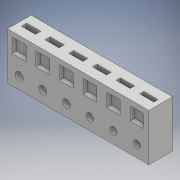
# Autodesk Inventor part: TOLERANCE_TEST
Saved by Autodesk Inventor 2017 (Build 210142000, 142)
## iProperties
Created: 2018-02-02
Part Number: TOLERANCE_TEST
Material: Generic
Document SubType Name: Modeling
Designer: Alex
Density: 1 g/cm^3
Appearance: Default
Author: Alex
Autodesk Inventor part; units mm, degrees
ref_plane "YZ Plane" through (0, 0, 0) normal (1, 0, 0) x (0, 1, 0)
ref_plane "XZ Plane" through (0, 0, 0) normal (0, 1, 0) x (-1, 0, 0)
ref_plane "XY Plane" through (0, 0, 0) normal (0, 0, 1) x (1, 0, 0)
sketch "Sketch1" plane through (0, 0, 0) normal (0, 1, 0) x (-1, 0, 0)
  line L0 (-30, 10) -> (30, 10)
  line L1 (30, 10) -> (30, -10)
  line L2 (30, -10) -> (-30, -10)
  line L3 (-30, -10) -> (-30, 10)
  point P0 (0, 0)
  point P1 (30, 0)
  point P2 (0, 10)
  dimension "d0" = 60
  dimension "d1" = 20
  constraints: 8 end point, 2 midpoint, 2 parallel, 1 horizontal, 1 horizontal alignment, 1 perpendicular, 1 vertical alignment
  measures "d0" distance of L0.start L0.end
  measures "d1" distance of L2.end L0.start
extrude "Extrusion1" add sketch "Sketch1" along normal blind 10
sketch "Sketch2" plane through (0, 10, 0) normal (0, 1, 0) x (1, 0, 0)
  line L0 (27.75, -7.75) -> (22.25, -7.75)
  line L1 (22.25, -7.75) -> (22.25, -2.25)
  line L2 (22.25, -2.25) -> (27.75, -2.25)
  line L3 (27.75, -2.25) -> (27.75, -7.75)
  line L4 (30, -10) -> (30, 10) projected
  line L5 (-30, -10) -> (30, -10) projected
  line L6 (12.2, -7.8) -> (17.8, -7.8)
  line L7 (17.8, -7.8) -> (17.8, -2.2)
  line L8 (17.8, -2.2) -> (12.2, -2.2)
  line L9 (12.2, -2.2) -> (12.2, -7.8)
  line L10 (2.15, -7.85) -> (7.85, -7.85)
  line L11 (7.85, -7.85) -> (7.85, -2.15)
  line L12 (7.85, -2.15) -> (2.15, -2.15)
  line L13 (2.15, -2.15) -> (2.15, -7.85)
  line L14 (-7.9, -7.9) -> (-2.1, -7.9)
  line L15 (-2.1, -7.9) -> (-2.1, -2.1)
  line L16 (-2.1, -2.1) -> (-7.9, -2.1)
  line L17 (-7.9, -2.1) -> (-7.9, -7.9)
  line L18 (-17.95, -7.95) -> (-12.05, -7.95)
  line L19 (-12.05, -7.95) -> (-12.05, -2.05)
  line L20 (-12.05, -2.05) -> (-17.95, -2.05)
  line L21 (-17.95, -2.05) -> (-17.95, -7.95)
  line L22 (-28, -8) -> (-22, -8)
  line L23 (-22, -8) -> (-22, -2)
  line L24 (-22, -2) -> (-28, -2)
  line L25 (-28, -2) -> (-28, -8)
  point P0 (0, 0)
  point P1 (-12.05, -5)
  point P2 (-7.9, -5)
  point P3 (-2.1, -5)
  point P4 (2.15, -5)
  point P5 (7.85, -5)
  point P6 (12.2, -5)
  point P7 (17.8, -5)
  point P8 (22.25, -5)
  point P9 (15, -7.8)
  point P10 (25, -7.75)
  point P11 (5, -7.85)
  point P12 (-5, -7.9)
  point P13 (-15, -7.95)
  point P14 (-25, -8)
  point P15 (-22, -5)
  point P16 (-17.95, -5)
  dimension "d9" = 5.5
  dimension "d10" = 5.6
  dimension "d11" = 5.7
  dimension "d12" = 5.8
  dimension "d13" = 5.9
  dimension "d14" = 10
  dimension "d15" = 10
  dimension "d16" = 10
  dimension "d17" = 10
  dimension "d18" = 5
  dimension "d19" = 6
  dimension "d20" = 10
  dimension "d65" = 5
  constraints: 48 end point, 16 midpoint, 12 parallel, 12 perpendicular, 6 horizontal, 5 horizontal alignment
  measures "d9" distance of L1.end L2.end
  measures "d10" distance of L7.end L8.end
  measures "d11" distance of L11.end L12.end
  measures "d12" distance of L15.end L16.end
  measures "d13" distance of L19.end L20.end
  measures "d14" horizontal distance of point (25, -7.75) point (15, -7.8)
  measures "d15" horizontal distance of point (15, -7.8) point (5, -7.85)
  measures "d16" horizontal distance of point (5, -7.85) point (-5, -7.9)
  measures "d17" horizontal distance of point (-5, -7.9) point (-15, -7.95)
  measures "d18" distance from line of L4 point (25, -7.75)
  measures "d19" distance of L23.end L24.end
  measures "d20" horizontal distance of point (-25, -8) point (-15, -7.95)
  measures "d65" distance from line of L5 point (22.25, -5)
extrude "Extrusion2" cut sketch "Sketch2" against normal blind 1.8
sketch "Sketch3" plane through (-30, 0, 10) normal (0, 0, 1) x (1, 0, 0)
  line L0 (2, 6.15) -> (8, 6.15)
  line L1 (8, 6.15) -> (8, 3.85)
  line L2 (8, 3.85) -> (2, 3.85)
  line L3 (2, 3.85) -> (2, 6.15)
  line L4 (12, 6.1) -> (18, 6.1)
  line L5 (18, 6.1) -> (18, 3.9)
  line L6 (18, 3.9) -> (12, 3.9)
  line L7 (12, 3.9) -> (12, 6.1)
  line L8 (22, 6.05) -> (28, 6.05)
  line L9 (28, 6.05) -> (28, 3.95)
  line L10 (28, 3.95) -> (22, 3.95)
  line L11 (22, 3.95) -> (22, 6.05)
  line L12 (32, 6) -> (38, 6)
  line L13 (38, 6) -> (38, 4)
  line L14 (38, 4) -> (32, 4)
  line L15 (32, 4) -> (32, 6)
  line L16 (42, 5.95) -> (48, 5.95)
  line L17 (48, 5.95) -> (48, 4.05)
  line L18 (48, 4.05) -> (42, 4.05)
  line L19 (42, 4.05) -> (42, 5.95)
  line L20 (52, 5.9) -> (58, 5.9)
  line L21 (58, 5.9) -> (58, 4.1)
  line L22 (58, 4.1) -> (52, 4.1)
  line L23 (52, 4.1) -> (52, 5.9)
  line L24 (60, 0) -> (60, 10) projected
  point P0 (30, 0)
  point P1 (55, 5.9)
  point P2 (45, 5.95)
  point P3 (35, 6)
  point P4 (25, 6.05)
  point P5 (15, 6.1)
  point P6 (5, 6.15)
  point P7 (8, 5)
  point P8 (12, 5)
  point P9 (18, 5)
  point P10 (22, 5)
  point P11 (28, 5)
  point P12 (32, 5)
  point P13 (38, 5)
  point P14 (42, 5)
  point P15 (48, 5)
  point P16 (52, 5)
  point P17 (58, 5)
  point P18 (60, 5)
  dimension "d23" = 6
  dimension "d24" = 1.8
  dimension "d25" = 5
  dimension "d26" = 10
  dimension "d27" = 10
  dimension "d28" = 10
  dimension "d29" = 10
  dimension "d30" = 10
  dimension "d31" = 1.9
  dimension "d32" = 2
  dimension "d33" = 2.1
  dimension "d34" = 2.2
  dimension "d35" = 2.3
  constraints: 48 end point, 18 midpoint, 17 parallel, 6 horizontal, 6 horizontal alignment, 6 perpendicular
  measures "d23" distance of L20.start L20.end
  measures "d24" distance of L20.end L21.end
  measures "d25" distance from line of point (55, 5.9) L24
  measures "d26" horizontal distance of point (55, 5.9) point (45, 5.95)
  measures "d27" horizontal distance of point (45, 5.95) point (35, 6)
  measures "d28" horizontal distance of point (35, 6) point (25, 6.05)
  measures "d29" horizontal distance of point (25, 6.05) point (15, 6.1)
  measures "d30" horizontal distance of point (15, 6.1) point (5, 6.15)
  measures "d31" distance of L16.end L17.end
  measures "d32" distance of L12.end L13.end
  measures "d33" distance of L8.end L9.end
  measures "d34" distance of L4.end L5.end
  measures "d35" distance of L0.end L1.end
extrude "Extrusion3" cut sketch "Sketch3" against normal blind 6
sketch "Sketch4" plane through (0, 0, 0) normal (0, -1, 0) x (1, 0, 0)
  line L0 (27.75, 2.25) -> (22.25, 2.25)
  line L1 (22.25, 2.25) -> (22.25, 7.75)
  line L2 (22.25, 7.75) -> (27.75, 7.75)
  line L3 (27.75, 7.75) -> (27.75, 2.25)
  line L4 (12.2, 2.2) -> (17.8, 2.2)
  line L5 (17.8, 2.2) -> (17.8, 7.8)
  line L6 (17.8, 7.8) -> (12.2, 7.8)
  line L7 (12.2, 7.8) -> (12.2, 2.2)
  line L8 (2.15, 2.15) -> (7.85, 2.15)
  line L9 (7.85, 2.15) -> (7.85, 7.85)
  line L10 (7.85, 7.85) -> (2.15, 7.85)
  line L11 (2.15, 7.85) -> (2.15, 2.15)
  line L12 (-7.9, 2.1) -> (-2.1, 2.1)
  line L13 (-2.1, 2.1) -> (-2.1, 7.9)
  line L14 (-2.1, 7.9) -> (-7.9, 7.9)
  line L15 (-7.9, 7.9) -> (-7.9, 2.1)
  line L16 (-17.95, 2.05) -> (-12.05, 2.05)
  line L17 (-12.05, 2.05) -> (-12.05, 7.95)
  line L18 (-12.05, 7.95) -> (-17.95, 7.95)
  line L19 (-17.95, 7.95) -> (-17.95, 2.05)
  line L20 (-28, 2) -> (-22, 2)
  line L21 (-22, 2) -> (-22, 8)
  line L22 (-22, 8) -> (-28, 8)
  line L23 (-28, 8) -> (-28, 2)
  line L24 (30, 10) -> (-30, 10) projected
  line L25 (30, -10) -> (30, 10) projected
  point P0 (0, 0)
  point P1 (-12.05, 5)
  point P2 (-7.9, 5)
  point P3 (-2.1, 5)
  point P4 (2.15, 5)
  point P5 (7.85, 5)
  point P6 (12.2, 5)
  point P7 (17.8, 5)
  point P8 (22.25, 5)
  point P9 (15, 2.2)
  point P10 (25, 2.25)
  point P11 (5, 2.15)
  point P12 (-5, 2.1)
  point P13 (-15, 2.05)
  point P14 (-25, 2)
  point P15 (-22, 5)
  point P16 (-17.95, 5)
  dimension "d38" = 5.5
  dimension "d39" = 5.6
  dimension "d40" = 5.7
  dimension "d41" = 5.8
  dimension "d42" = 5.9
  dimension "d43" = 10
  dimension "d44" = 10
  dimension "d45" = 10
  dimension "d46" = 10
  dimension "d47" = 6
  dimension "d48" = 10
  dimension "d51" = 5
  dimension "d53" = 5
  constraints: 48 end point, 16 midpoint, 12 parallel, 12 perpendicular, 6 horizontal, 5 horizontal alignment
  measures "d38" distance of L2.start L2.end
  measures "d39" distance of L6.start L7.start
  measures "d40" distance of L10.start L11.start
  measures "d41" distance of L13.end L15.start
  measures "d42" distance of L17.end L18.end
  measures "d43" horizontal distance of point (25, 2.25) point (15, 2.2)
  measures "d44" horizontal distance of point (15, 2.2) point (5, 2.15)
  measures "d45" horizontal distance of point (5, 2.15) point (-5, 2.1)
  measures "d46" horizontal distance of point (-5, 2.1) point (-15, 2.05)
  measures "d47" distance of L21.end L22.end
  measures "d48" horizontal distance of point (-25, 2) point (-15, 2.05)
  measures "d51" distance from line of L24 point (22.25, 5)
  measures "d53" distance from line of L25 point (25, 2.25)
extrude "Extrusion4" cut sketch "Sketch4" against normal blind 1.8
hole "Hole1" at (25, 10, -5) direction (0, -1, 0) diameter 3 end through all counterbore diameter 5.5 counterbore depth 3
hole "Hole2" at (15, 10, -5) direction (0, -1, 0) diameter 3.1 end through all counterbore diameter 5.6 counterbore depth 3.1
hole "Hole3" at (5, 10, -5) direction (0, -1, 0) diameter 3.2 end through all counterbore diameter 5.7 counterbore depth 3.2
hole "Hole4" at (-5, 10, -5) direction (0, -1, 0) diameter 3.3 end through all counterbore diameter 5.8 counterbore depth 3.3
hole "Hole5" at (-15, 10, -5) direction (0, -1, 0) diameter 3.4 end through all counterbore diameter 5.9 counterbore depth 3.4
hole "Hole6" at (-25, 10, -5) direction (0, -1, 0) diameter 3.5 end through all counterbore diameter 6 counterbore depth 3.5
equation "\"d9\" = nut_A"
equation "\"d21\" = nut_B"
equation "\"d24\" = nut_B"
equation "\"d38\" = d49"
equation "\"d54\" = nut_B"
equation "\"d58\" = screw_m3_A"
equation "\"d60\" = screw_m3_C"
equation "\"d61\" = screw_m3_D"
equation "\"nut_A\" = 5.5"
equation "\"nut_B\" = 1.8"
equation "\"d49\" = 5.5"
equation "\"screw_m3_A\" = 3"
equation "\"screw_m3_C\" = 5.5"
equation "\"screw_m3_D\" = 3"
body "Solid1"
